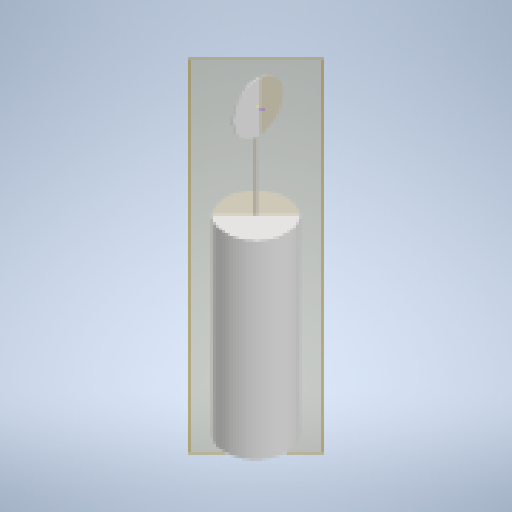
# Autodesk Inventor part: CRS4kHz
Saved by Autodesk Inventor 2024.2 (Build 282272000, 272)
## iProperties
Created: 2021-07-18
Part Number: CRS4kHz
Material: Generic
Document SubType Name: Modeling
Designer: MicroscopyInnovation
Density: 1 g/cm^3
Appearance: Default
Author: MicroscopyInnovation
Autodesk Inventor part; units mm, degrees
ref_plane "YZ Plane" through (0, 0, 0) normal (1, 0, 0) x (0, 1, 0)
ref_plane "XZ Plane" through (0, 0, 0) normal (0, 1, 0) x (-1, 0, 0)
sketch "Sketch1" plane through (0, 0, 0) normal (0, 1, 0) x (-1, 0, 0)
  circle A0 centre (0, 0) radius 7.9375
  dimension "d0" = 15.875
  constraints: 1 centre point, 1 coincident
  measures "d0" diameter of A0
extrude "Extrusion1" add sketch "Sketch1" along normal blind 48.895
sketch "Sketch2" plane through (0, 48.895, 0) normal (0, 1, 0) x (1, 0, 0)
  circle A0 centre (0, 0) radius 0.2794
  dimension "d3" = 0.5588
  constraints: 1 centre point, 1 coincident
  measures "d3" diameter of A0
extrude "Extrusion2" add sketch "Sketch2" along normal blind 24.384
sketch "Sketch3" plane through (0, 73.279, 0) normal (0, 1, 0) x (1, 0, 0)
  circle A0 centre (0, 0) radius 0.2794 projected
  point P0 (0.2794, 0)
  constraints: 1 horizontal alignment, 1 other
ref_plane "Work Plane1" through (0.2794, 73.279, 0) normal (1, 0, 0) x (0, 1, 0)
sketch "Sketch4" plane through (0.2794, 73.279, 0) normal (1, 0, 0) x (0, 1, 0)
  line L0 (0, -0.2794) -> (0, 0.2794) projected
  circle A0 centre (0, 0) radius 6.3754
  point P0 (-73.279, 0)
  dimension "d6" = 12.7508
  constraints: 1 centre point, 1 midpoint
  measures "d6" diameter of A0
extrude "Extrusion3" add sketch "Sketch4" along normal blind 0.2794
ref_plane "Work Plane4" through (0, 73.279, 0) normal (0.7071, 0, 0.7071) x (0, -1, 0)
ref_plane "Work Plane3" through (0.5588, 73.279, 0) normal (0.7071, 0, 0.7071) x (0, -1, 0)
body "Solid1"
